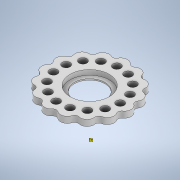
# Autodesk Inventor part: Rotor
Saved by Autodesk Inventor 2021 (Build 250183000, 183)
## iProperties
Created: 2022-07-10
Part Number: Rotor
Material: Ogólny
Document SubType Name: Modeling
Designer: MicnedSQ
Density: 1 g/cm^3
Appearance: Domyślna
Author: MicnedSQ
## iProperties of the stored document _Drukowanie 3D.ipt
Created: 2022-08-06
Part Number: _Drukowanie 3D
Material: Ogólny
Document SubType Name: Modeling
Designer: MicnedSQ
Density: 1 g/cm^3
Appearance: Domyślna
Author: MicnedSQ
Autodesk Inventor part; units mm, degrees
ref_plane "YZ Plane" through (0, 0, 0) normal (1, 0, 0) x (0, 1, 0)
ref_plane "XZ Plane" through (0, 0, 0) normal (0, 1, 0) x (-1, 0, 0)
ref_plane "XY Plane" through (0, 0, 0) normal (0, 0, 1) x (1, 0, 0)
sketch "Szkic3" plane through (0, 0, 0) normal (0, 1, 0) x (-1, 0, 0)
  spline S0 degree 5 poles (31, 0) (31.0002, -0.5578) (31.1372, -1.1146) (31.406, -1.6352) (32.007, -2.2538) (32.5316, -2.9419) (32.6959, -3.2013) (33.0392, -3.8571) (33.2567, -4.5662) (33.3404, -4.993) (33.4301, -5.9129) (33.3333, -6.8338) (33.231, -7.3149) (32.9449, -8.1955) (32.4888, -8.9994) (32.2388, -9.3553) (31.7516, -9.9146) (31.1713, -10.3741) (30.9157, -10.5443) (30.1566, -10.9594) (29.3557, -11.2803) (28.899, -11.6461) (28.1944, -12.5529) (27.9919, -13.6834) (28.0257, -14.2675) (28.3231, -15.0775) (28.5226, -15.9193) (28.5671, -16.2231) (28.6139, -16.9618) (28.5243, -17.6982) (28.4271, -18.1221) (28.1349, -18.999) (27.6719, -19.8008) (27.3828, -20.1987) (26.7633, -20.8868) (26.0196, -21.4358) (25.6464, -21.6592) (24.9739, -21.972) (24.2569, -22.1557) (23.9541, -22.2072) (23.0919, -22.2777) (22.2296, -22.2451) (21.6636, -22.3935) (20.6511, -22.9354) (20.0064, -23.8857) (19.7996, -24.4331) (19.7419, -25.294) (19.5817, -26.1442) (19.4988, -26.4399) (19.2411, -27.1337) (18.8598, -27.77) (18.5986, -28.1177) (17.9749, -28.7999) (17.2258, -29.3441) (16.7999, -29.59) (15.954, -29.9667) (15.0514, -30.1657) (14.6196, -30.218) (13.8779, -30.2302) (13.1482, -30.1064) (12.8507, -30.0303) (12.0343, -29.744) (11.2599, -29.3635) (10.6825, -29.2689) (9.5371, -29.3521) (8.5615, -29.958) (8.15, -30.374) (7.7471, -31.137) (7.255, -31.8485) (7.059, -32.0849) (6.5414, -32.614) (5.9342, -33.0401) (5.5541, -33.2515) (4.7069, -33.6211) (3.8012, -33.8136) (3.3121, -33.865) (2.3862, -33.865) (1.4806, -33.6797) (1.0649, -33.5518) (0.3824, -33.2613) (-0.2339, -32.8514) (-0.4748, -32.6609) (-1.1041, -32.0673) (-1.6568, -31.4047) (-2.1458, -31.0834) (-3.226, -30.6935) (-4.3637, -30.8503) (-4.9088, -31.0629) (-5.5872, -31.5961) (-6.3262, -32.0459) (-6.6014, -32.1822) (-7.2895, -32.455) (-8.0175, -32.5972) (-8.4507, -32.6359) (-9.375, -32.6289) (-10.2806, -32.4363) (-10.7484, -32.2843) (-11.5943, -31.9078) (-12.3461, -31.3701) (-12.6739, -31.0843) (-13.1793, -30.5413) (-13.5756, -29.9161) (-13.7181, -29.6441) (-14.0516, -28.8458) (-14.287, -28.0158) (-14.6031, -27.5233) (-15.4313, -26.7278) (-16.5344, -26.4083) (-17.1188, -26.3808) (-17.9554, -26.592) (-18.8135, -26.7023) (-19.1203, -26.7148) (-19.8599, -26.6842) (-20.5828, -26.5181) (-20.9943, -26.3771) (-21.8358, -25.9948) (-22.5849, -25.4505) (-22.9504, -25.1215) (-23.5699, -24.4334) (-24.0381, -23.6364) (-24.2213, -23.2419) (-24.4621, -22.5403) (-24.5699, -21.8081) (-24.5895, -21.5016) (-24.5694, -20.6367) (-24.4469, -19.7826) (-24.5353, -19.2042) (-24.9684, -18.1406) (-25.8461, -17.4) (-26.3689, -17.1372) (-27.219, -16.9898) (-28.0478, -16.7416) (-28.3332, -16.6283) (-28.9963, -16.2995) (-29.5892, -15.8537) (-29.9078, -15.5576) (-30.521, -14.866) (-30.984, -14.0641) (-31.184, -13.6148) (-31.4702, -12.7342) (-31.5737, -11.8158) (-31.5806, -11.3809) (-31.5152, -10.642) (-31.3158, -9.9292) (-31.2091, -9.6412) (-30.839, -8.8593) (-30.3797, -8.1289) (-30.2252, -7.5645) (-30.1882, -6.4167) (-30.6888, -5.3832) (-31.0595, -4.9304) (-31.7762, -4.45) (-32.4324, -3.8862) (-32.647, -3.6665) (-33.1191, -3.0965) (-33.4794, -2.448) (-33.6499, -2.048) (-33.9289, -1.1668) (-34.0257, -0.2459) (-34.0257, 0.2459) (-33.9289, 1.1668) (-33.6499, 2.048) (-33.4794, 2.448) (-33.1191, 3.0965) (-32.647, 3.6665) (-32.4324, 3.8862) (-31.7762, 4.45) (-31.0595, 4.9304) (-30.6888, 5.3832) (-30.1882, 6.4167) (-30.2252, 7.5645) (-30.3797, 8.1289) (-30.839, 8.8593) (-31.2091, 9.6412) (-31.3158, 9.9292) (-31.5152, 10.642) (-31.5806, 11.3809) (-31.5737, 11.8158) (-31.4702, 12.7342) (-31.184, 13.6148) (-30.984, 14.0641) (-30.521, 14.866) (-29.9078, 15.5576) (-29.5892, 15.8537) (-28.9963, 16.2995) (-28.3332, 16.6283) (-28.0478, 16.7416) (-27.219, 16.9898) (-26.3689, 17.1372) (-25.8461, 17.4) (-24.9684, 18.1406) (-24.5353, 19.2042) (-24.4469, 19.7826) (-24.5694, 20.6367) (-24.5895, 21.5016) (-24.5699, 21.8081) (-24.4621, 22.5403) (-24.2213, 23.2419) (-24.0381, 23.6364) (-23.5699, 24.4334) (-22.9504, 25.1215) (-22.5849, 25.4505) (-21.8358, 25.9948) (-20.9943, 26.3771) (-20.5828, 26.5181) (-19.8599, 26.6842) (-19.1203, 26.7148) (-18.8135, 26.7023) (-17.9554, 26.592) (-17.1188, 26.3808) (-16.5344, 26.4083) (-15.4313, 26.7278) (-14.6031, 27.5233) (-14.287, 28.0158) (-14.0516, 28.8458) (-13.7181, 29.6441) (-13.5756, 29.9161) (-13.1793, 30.5413) (-12.6739, 31.0843) (-12.3461, 31.3701) (-11.5943, 31.9078) (-10.7484, 32.2843) (-10.2806, 32.4363) (-9.375, 32.6289) (-8.4507, 32.6359) (-8.0175, 32.5972) (-7.2895, 32.455) (-6.6014, 32.1822) (-6.3262, 32.0459) (-5.5872, 31.5961) (-4.9088, 31.0629) (-4.3637, 30.8503) (-3.226, 30.6935) (-2.1458, 31.0834) (-1.6568, 31.4047) (-1.1041, 32.0673) (-0.4748, 32.6609) (-0.2339, 32.8514) (0.3824, 33.2613) (1.0649, 33.5518) (1.4806, 33.6797) (2.3862, 33.865) (3.3121, 33.865) (3.8012, 33.8136) (4.7069, 33.6211) (5.5541, 33.2515) (5.9342, 33.0401) (6.5414, 32.614) (7.059, 32.0849) (7.255, 31.8485) (7.7471, 31.137) (8.15, 30.374) (8.5615, 29.958) (9.5371, 29.3521) (10.6825, 29.2689) (11.2599, 29.3635) (12.0343, 29.744) (12.8507, 30.0303) (13.1482, 30.1064) (13.8779, 30.2302) (14.6196, 30.218) (15.0514, 30.1657) (15.954, 29.9667) (16.7999, 29.59) (17.2258, 29.3441) (17.9749, 28.7999) (18.5986, 28.1177) (18.8598, 27.77) (19.2411, 27.1337) (19.4988, 26.4399) (19.5817, 26.1442) (19.7419, 25.294) (19.7996, 24.4331) (20.0064, 23.8857) (20.6511, 22.9354) (21.6636, 22.3935) (22.2296, 22.2451) (23.0919, 22.2777) (23.9541, 22.2072) (24.2569, 22.1557) (24.9739, 21.972) (25.6464, 21.6592) (26.0196, 21.4358) (26.7633, 20.8868) (27.3828, 20.1987) (27.6719, 19.8008) (28.1349, 18.999) (28.4271, 18.1221) (28.5243, 17.6982) (28.6139, 16.9618) (28.5671, 16.2231) (28.5226, 15.9193) (28.3231, 15.0775) (28.0257, 14.2675) (27.9919, 13.6834) (28.1944, 12.5529) (28.899, 11.6461) (29.3557, 11.2803) (30.1566, 10.9594) (30.9157, 10.5443) (31.1713, 10.3741) (31.7516, 9.9146) (32.2388, 9.3553) (32.4888, 8.9994) (32.9449, 8.1955) (33.231, 7.3149) (33.3333, 6.8338) (33.4301, 5.9129) (33.3404, 4.993) (33.2567, 4.5662) (33.0392, 3.8571) (32.6959, 3.2013) (32.5316, 2.9419) (32.007, 2.2538) (31.406, 1.6352) (31.1372, 1.1146) (31.0002, 0.5578) (31, 0) knots 0 0 0 0 0 0 0.012068 0.012068 0.012068 0.018691 0.018691 0.018691 0.028044 0.028044 0.028044 0.038623 0.038623 0.038623 0.047975 0.047975 0.047975 0.054598 0.054598 0.054598 0.066667 0.066667 0.066667 0.078735 0.078735 0.078735 0.085358 0.085358 0.085358 0.09471 0.09471 0.09471 0.10529 0.10529 0.10529 0.114642 0.114642 0.114642 0.121265 0.121265 0.121265 0.133333 0.133333 0.133333 0.145402 0.145402 0.145402 0.152025 0.152025 0.152025 0.161377 0.161377 0.161377 0.171956 0.171956 0.171956 0.181309 0.181309 0.181309 0.187932 0.187932 0.187932 0.2 0.2 0.2 0.212068 0.212068 0.212068 0.218691 0.218691 0.218691 0.228044 0.228044 0.228044 0.238623 0.238623 0.238623 0.247975 0.247975 0.247975 0.254598 0.254598 0.254598 0.266667 0.266667 0.266667 0.278735 0.278735 0.278735 0.285358 0.285358 0.285358 0.29471 0.29471 0.29471 0.30529 0.30529 0.30529 0.314642 0.314642 0.314642 0.321265 0.321265 0.321265 0.333333 0.333333 0.333333 0.345402 0.345402 0.345402 0.352025 0.352025 0.352025 0.361377 0.361377 0.361377 0.371956 0.371956 0.371956 0.381309 0.381309 0.381309 0.387932 0.387932 0.387932 0.4 0.4 0.4 0.412068 0.412068 0.412068 0.418691 0.418691 0.418691 0.428044 0.428044 0.428044 0.438623 0.438623 0.438623 0.447975 0.447975 0.447975 0.454598 0.454598 0.454598 0.466667 0.466667 0.466667 0.478735 0.478735 0.478735 0.485358 0.485358 0.485358 0.49471 0.49471 0.49471 0.50529 0.50529 0.50529 0.514642 0.514642 0.514642 0.521265 0.521265 0.521265 0.533333 0.533333 0.533333 0.545402 0.545402 0.545402 0.552025 0.552025 0.552025 0.561377 0.561377 0.561377 0.571956 0.571956 0.571956 0.581309 0.581309 0.581309 0.587932 0.587932 0.587932 0.6 0.6 0.6 0.612068 0.612068 0.612068 0.618691 0.618691 0.618691 0.628044 0.628044 0.628044 0.638623 0.638623 0.638623 0.647975 0.647975 0.647975 0.654598 0.654598 0.654598 0.666667 0.666667 0.666667 0.678735 0.678735 0.678735 0.685358 0.685358 0.685358 0.69471 0.69471 0.69471 0.70529 0.70529 0.70529 0.714642 0.714642 0.714642 0.721265 0.721265 0.721265 0.733333 0.733333 0.733333 0.745402 0.745402 0.745402 0.752025 0.752025 0.752025 0.761377 0.761377 0.761377 0.771956 0.771956 0.771956 0.781309 0.781309 0.781309 0.787932 0.787932 0.787932 0.8 0.8 0.8 0.812068 0.812068 0.812068 0.818691 0.818691 0.818691 0.828044 0.828044 0.828044 0.838623 0.838623 0.838623 0.847975 0.847975 0.847975 0.854598 0.854598 0.854598 0.866667 0.866667 0.866667 0.878735 0.878735 0.878735 0.885358 0.885358 0.885358 0.89471 0.89471 0.89471 0.90529 0.90529 0.90529 0.914642 0.914642 0.914642 0.921265 0.921265 0.921265 0.933333 0.933333 0.933333 0.945402 0.945402 0.945402 0.952025 0.952025 0.952025 0.961377 0.961377 0.961377 0.971956 0.971956 0.971956 0.981309 0.981309 0.981309 0.987932 0.987932 0.987932 1 1 1 1 1 1
  circle A0 centre (-25, 0) radius 3.25
  circle A1 centre (-22.8386, -10.1684) radius 3.25
  circle A2 centre (-16.7283, -18.5786) radius 3.25
  circle A3 centre (-7.7254, -23.7764) radius 3.25
  circle A4 centre (2.6132, -24.863) radius 3.25
  circle A5 centre (12.5, -21.6506) radius 3.25
  circle A6 centre (20.2254, -14.6946) radius 3.25
  circle A7 centre (24.4537, -5.1978) radius 3.25
  circle A8 centre (24.4537, 5.1978) radius 3.25
  circle A9 centre (20.2254, 14.6946) radius 3.25
  circle A10 centre (12.5, 21.6506) radius 3.25
  circle A11 centre (2.6132, 24.863) radius 3.25
  circle A12 centre (-7.7254, 23.7764) radius 3.25
  circle A13 centre (-16.7283, 18.5786) radius 3.25
  circle A14 centre (-22.8386, 10.1684) radius 3.25
  circle A15 centre (0, 0) radius 12.5
  point P0 (36, 0)
  dimension "d16" = 6.5
  dimension "d19" = 360
  dimension "d21" = 25
  dimension "d22" = 25
  constraints: 16 centre point, 1 coincident, 33 other
  measures "d16" diameter of A0
  measures "d21" distance of A0.centre point (0, 0)
  measures "d22" diameter of A15
extrude "Wyciągnięcie proste1" add sketch "Szkic3" along normal blind 5
sketch "Szkic4" plane through (0, 5, 0) normal (0, 1, 0) x (1, 0, 0)
  circle A0 centre (0, 0) radius 16
  dimension "d25" = 32
  constraints: 1 centre point, 1 coincident
  measures "d25" diameter of A0
extrude "Wyciągnięcie proste2" cut sketch "Szkic4" against normal blind 4
equation "curve S0 of \"Szkic3\": x = (35*cos(t))-(2.5*cos(t+atan(sin((1-16)*t)/((35/1.5/16)-cos((1-16)*t)))))-(1.5*cos(16*t)); y = (-35*sin(t))+(2.5*sin(t+atan(sin((1-16)*t)/((35/1.5/16)-cos((1-16)*t)))))+(1.5*s"
